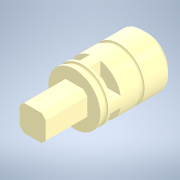
# Autodesk Inventor part: VacuumRotor
Saved by Autodesk Inventor 2020 (Build 240168000, 168)
## iProperties
Created: 2020-03-07
Part Number: VacuumRotor
Material: Nylon, molybdenum disulphide
Document SubType Name: Modeling
Designer: 10300812
Density: 1.13 g/cm^3
Appearance: Nylon 6
Author: 10300812
Autodesk Inventor part; units mm, degrees
ref_plane "YZ Plane" through (0, 0, 0) normal (1, 0, 0) x (0, 1, 0)
ref_plane "XZ Plane" through (0, 0, 0) normal (0, 1, 0) x (-1, 0, 0)
ref_plane "XY Plane" through (0, 0, 0) normal (0, 0, 1) x (1, 0, 0)
sketch "Sketch1" plane through (0, 0, 0) normal (0, 0, 1) x (1, 0, 0)
  circle A0 centre (0, 0) radius 2.5
  circle A1 centre (0, 0) radius 5
  dimension "d0" = 5
  dimension "d1" = 10
  constraints: 2 centre point, 2 coincident
  measures "d0" diameter of A0
  measures "d1" diameter of A1
extrude "Extrusion1" add sketch "Sketch1" along normal blind 10
sketch "Sketch2" plane through (0, 0, 10) normal (0, 0, 1) x (1, 0, 0)
  circle A0 centre (0, 0) radius 5 projected
  circle A1 centre (0, 0) radius 5 projected
  line L0 (-4.899, 1) -> (4.899, 1)
  line L1 (-4.899, -1) -> (4.899, -1)
  line L2 (-1, 4.899) -> (-1, -4.899)
  line L3 (1, -4.899) -> (1, 4.899)
  point P0 (1, 1)
  point P1 (-1, 1)
  point P2 (-1, -1)
  point P3 (1, -1)
  dimension "d4" = 1
  dimension "d5" = 1
  dimension "d6" = 1
  dimension "d7" = 1
  constraints: 8 end point, 2 perpendicular, 1 horizontal, 1 parallel, 9 other
  measures "d4" distance from line of L0 point (0, 0)
  measures "d5" distance from line of point (0, 0) L1
  measures "d6" distance from line of point (0, 0) L2
  measures "d7" distance from line of L3 point (0, 0)
extrude "Extrusion2" add sketch "Sketch2" along normal blind 2 contours A0 L1 L3 L0 | L3 L0 L2 A0 | L3 L1 L2 L0 | A0 L2 L1 L3 | L2 L1 A0 L0
sketch "Sketch3" plane through (0, 0, 12) normal (0, 0, 1) x (1, 0, 0)
  circle A0 centre (0, 0) radius 5
  dimension "d11" = 10
  constraints: 1 centre point, 1 coincident
  measures "d11" diameter of A0
extrude "Extrusion3" add sketch "Sketch3" along normal blind 2
chamfer "Chamfer1" distance 1 angle 45 1 edges at (-5, 0, 0)
sketch "Sketch4" plane through (0, 0, 10) normal (0, 0, -1) x (-1, 0, 0)
  circle A0 centre (0, 0) radius 2
  dimension "d17" = 4
  constraints: 1 centre point, 1 coincident
  measures "d17" diameter of A0
extrude "Extrusion4" cut sketch "Sketch4" against normal blind 2
fillet "Fillet2" radius 0.5 8 edges at (-1, 1.7321, 11) (-1, -1.7321, 11) (-1.7321, -1, 11) (1.7321, -1, 11) (1.7321, 1, 11) (-1.7321, 1, 11) (1, 1.7321, 11) (1, -1.7321, 11)
sketch "Sketch5" plane through (0, 0, 14) normal (0, 0, 1) x (1, 0, 0)
  line L0 (-2.5, 2.5) -> (2.5, 2.5)
  line L1 (2.5, 2.5) -> (2.5, -2.5)
  line L2 (2.5, -2.5) -> (-2.5, -2.5)
  line L3 (-2.5, -2.5) -> (-2.5, 2.5)
  line L4 (-2.5, 2.5) -> (2.5, -2.5) construction
  line L5 (2.5, 2.5) -> (-2.5, -2.5) construction
  point P0 (0, 0)
  dimension "d21" = 5
  dimension "d22" = 5
  constraints: 12 end point, 2 midpoint, 2 parallel, 1 horizontal, 1 perpendicular
  measures "d21" distance of L1.end L2.end
  measures "d22" distance of L0.end L1.end
extrude "Extrusion5" add sketch "Sketch5" along normal blind 8
chamfer "Chamfer2" distance 0.8 angle 45 4 edges at (2.5, 2.5, 18) (-2.5, 2.5, 18) (2.5, -2.5, 18) (-2.5, -2.5, 18)
sketch "Sketch6" plane through (0, 0, 0) normal (1, 0, 0) x (0, 1, 0)
  line L0 (5.5, 13.5) -> (4.5, 13.5)
  line L1 (4.5, 13.5) -> (4.5, 12.5)
  line L2 (4.5, 12.5) -> (5.5, 12.5)
  line L3 (5.5, 12.5) -> (5.5, 13.5)
  line L4 (5, 1) -> (5, 14) projected
  line L5 (5.5, 13.5) -> (4.5, 12.5) construction
  line L6 (4.5, 13.5) -> (5.5, 12.5) construction
  line L7 (5.5, 6.5) -> (4.5, 6.5)
  line L8 (4.5, 6.5) -> (4.5, 5.5)
  line L9 (4.5, 5.5) -> (5.5, 5.5)
  line L10 (5.5, 5.5) -> (5.5, 6.5)
  line L11 (5.5, 6.5) -> (4.5, 5.5) construction
  line L12 (4.5, 6.5) -> (5.5, 5.5) construction
  line L13 (4.899, 10) -> (4.899, 12) projected
  line L14 (4.899, 12) -> (1, 12) projected
  line L15 (4.899, 12) -> (4.899, 14)
  line L16 (4.899, 10) -> (1, 10) projected
  line L17 (0, -4.4) -> (0, 26.4) projected
  point P0 (0, 0)
  point P1 (5, 13)
  point P2 (5, 6)
  dimension "d28" = 1
  dimension "d29" = 1
  dimension "d30" = 1
  dimension "d31" = 4
  constraints: 26 end point, 4 midpoint, 4 parallel, 2 horizontal, 2 perpendicular, 2 point on line, 1 collinear, 1 vertical, 1 vertical alignment
  measures "d28" distance of L9.end L7.start
  measures "d29" distance of L7.start L7.end
  measures "d30" distance of L4.end point (5, 13)
  measures "d31" distance from line of L16 point (5, 6)
revolve "Revolution1" cut sketch "Sketch6" angle 360 about axis through (0, 0, -10) along (0, 0, 1)
fillet "Fillet3" radius 0.4 4 edges at (0, -4.5, 13.5) (0, -4.5, 6.5) (0, -4.5, 5.5) (0, -4.5, 12.5)
equation "\"d5\" = d4"
equation "\"d6\" = d4"
body "Solid1"
